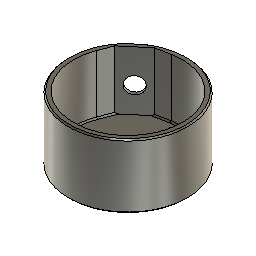
Gauge (Autodesk Fusion 360 design; units mm, degrees)
Autodesk Fusion 360 part; units mm, degrees
sketch "Sketch1" plane through (0, 0, 0) normal (0, 0, 1) x (1, 0, 0)
  circle A0 centre (0, 0) radius 42.5
  circle A1 centre (0, 0) radius 46.5
  dimension "d1" = 85
  dimension "d2" = 93
  constraint coincident A0.centre A1.centre
  constraint concentric A0 A1
  measures "d1" diameter of A0
  measures "d2" diameter of A1
extrude "Extrude1" add sketch "Sketch1" along normal blind 46 makes body 1
extrude "Extrude2" add sketch "Sketch1" against normal blind 4 contours A0 | A1 bodies 1
ref_plane "WorkPlane1" through (0, 0, 46) normal (0, 0, 1) x (1, 0, 0)
sketch "Sketch3" plane through (0, 0, 46) normal (0, 0, 1) x (1, 0, 0)
  circle A0 centre (0, 0) radius 46.5
  circle A1 centre (0, 0) radius 42.5
  circle A2 centre (0, 0) radius 49
  circle A3 centre (0, 0) radius 40.5
  circle A4 centre (0, 0) radius 46.9
  dimension "d9" = 98
  dimension "d10" = 81
  dimension "d50" = 0.4
  constraint concentric A0 A2
  constraint concentric A0 A3
  measures "d9" diameter of A2
  measures "d10" diameter of A3
extrude "Extrude3" add sketch "Sketch3" along normal blind 4 separate body contours A0 | A1 | A2 | A4 makes body 2
extrude "Extrude4" add sketch "Sketch3" against normal blind 12 contours A2 bodies 2
chamfer "Chamfer1" distance 3 angle 45 1 edges at (-37.7593, 14.6454, 50) on bodies 2
chamfer "Chamfer2" distance 2 angle 65 1 edges at (-45.684, -17.7192, 50) measured on face at (46.8223, -4.5955, 50) on bodies 2
chamfer "Chamfer3" distance 1 angle 45 1 edges at (-45.684, 17.7192, 34) measured on face at (48.1176, -2.4344, 34) on bodies 2
chamfer "Chamfer4" distance 1 angle 45 1 edges at (-43.3532, 16.8151, -4) measured on face at (10.204, -8.5364, -4) on bodies 1
ref_plane "WorkPlane2" through (0, 0, 0) normal (0, 0, -1) x (-1, 0, 0)
sketch "Sketch4" plane through (0, 0, 0) normal (0, 0, -1) x (1, 0, 0)
  circle A0 centre (0, 0) radius 46.5 construction
  line L0 (-37.4678, -27.5394) -> (-20.6148, -41.6807)
  line L1 (-20.6148, -41.6807) -> (-26.0712, -48.1834)
  line L2 (-26.0712, -48.1834) -> (-42.9242, -34.0421)
  line L3 (-42.9242, -34.0421) -> (-37.4678, -27.5394)
  line L4 (0, 0) -> (-58.0825, -69.2201) construction
  line L5 (-18.892, -39.6276) -> (-35.745, -25.4862)
  circle A1 centre (0, 0) radius 42.5
  line L6 (-18.892, -39.6276) -> (-8.0933, -41.7223)
  line L7 (-35.745, -25.4862) -> (-39.683, -15.2153)
  line L8 (-39.683, -15.2153) -> (-8.0933, -41.7223)
  line L9 (0, 0) -> (-65, 0) construction
  dimension "d26" = 22
  dimension "d58" = 50
  constraint coincident A0 L0.start
  constraint coincident A0 L0.end
  constraint coincident A0.centre L4.start
  constraint midpoint L0 L4
  constraint perpendicular L4 L5
  constraint tangent L5 A1
  constraint coincident A1 L6.end
  constraint coincident A1 L7.end
  constraint tangent A1 L6
  constraint tangent A1 L7
  constraint perpendicular L0 L3
  constraint perpendicular L0 L1
  constraint parallel L0 L2
  constraint horizontal L9
  constraint coincident L3 L5.end
  constraint coincident L1 L5.start
  measures "d26" distance of L0.start L0.end
  measures "d58" angle of L4 L9
extrude "Extrude5" cut sketch "Sketch4" along normal through all and the other way through all contours L0 L1 L2 L3 bodies 1
sketch "Sketch5" plane through (-29.0413, 34.61, 0) normal (-0.642788, 0.766044, 0) x (-0.766044, -0.642788, 0)
  line L0 (-11, 46) -> (-11, -3)
  circle A0 centre (0, 20) radius 6.5
  line L1 (11, 46) -> (-11, 46)
  spline S0 degree 2 poles (-5.3852, -4) (-8.1621, -3.6713) (-11, -3) knots 0 0 0 0.570553 0.570553 0.570553 weights 1 1.001868 1
  line L2 (-5.3852, -4) -> (5.3852, -4)
  spline S1 degree 2 poles (11, -3) (8.1621, -3.6713) (5.3852, -4) knots 0 0 0 0.570553 0.570553 0.570553 weights 1 1.001868 1
  line L3 (11, -3) -> (11, 46)
  line L4 (-11, 0) -> (11, 0)
  dimension "d30" = 13
  dimension "d61" = 20
  dimension "d62" = 11
  measures "d30" diameter of A0
  measures "d61" distance of A0.centre L4
  measures "d62" distance of L0 A0.centre
extrude "Extrude6" cut sketch "Sketch5" against normal blind 15 contours A0 bodies 1
sketch "Sketch6" plane through (0, 0, 0) normal (0, 0, 1) x (-1, 0, 0)
  circle A0 centre (0, -35) radius 3
  circle A1 centre (30.31, 17.5) radius 3
  circle A2 centre (-30.31, 17.5) radius 3
  circle A3 centre (0, 0) radius 5
  circle A4 centre (0, 0) radius 42.5
  circle A5 centre (20, 0) radius 2.75
  line L0 (0, 0) -> (65, 0)
  circle A6 centre (-20, 0) radius 2.75
  circle A7 centre (20, 0) radius 5
  circle A8 centre (-20, 0) radius 5
  dimension "d33" = 6
  dimension "d34" = 6
  dimension "d35" = 6
  dimension "d36" = 35
  dimension "d37" = 17.5
  dimension "d38" = 17.5
  dimension "d39" = 30.31
  dimension "d40" = 30.31
  dimension "d42" = 10
  dimension "d63" = 5.5
  dimension "d64" = 5.5
  dimension "d65" = 10
  dimension "d66" = 10
  dimension "d67" = 20
  dimension "d68" = 20
  constraint vertical A3.centre A0.centre
  constraint coincident A3.centre A4.centre
  constraint coincident A5.centre L0
  constraint concentric A5 A7
  constraint concentric A6 A8
  constraint horizontal A3.centre A6.centre
  measures "d33" diameter of A1
  measures "d34" diameter of A2
  measures "d35" diameter of A0
  measures "d36" distance of A3.centre A0.centre
  measures "d37" vertical distance of A3.centre A1.centre
  measures "d38" vertical distance of A3.centre A2.centre
  measures "d39" horizontal distance of A3.centre A2.centre
  measures "d40" horizontal distance of A3.centre A1.centre
  measures "d42" diameter of A3
  measures "d63" diameter of A6
  measures "d64" diameter of A5
  measures "d65" diameter of A8
  measures "d66" diameter of A7
  measures "d67" distance of A3.centre A5.centre
  measures "d68" distance of A3.centre A6.centre
extrude "Extrude7" cut sketch "Sketch6" against normal through all contours A3 | A5 L0 | A5 L0 | A6 bodies 1
extrude "Extrude8" add sketch "Sketch6" along normal blind 2 contours A0 | A1 | A2 bodies 1
sketch "Sketch7" plane through (0, 0, 2) normal (0, 0, 1) x (-1, 0, 0)
  circle A0 centre (0, -35) radius 3
  circle A1 centre (0, -35) radius 1.5
  circle A2 centre (30.31, 17.5) radius 1.5
  circle A3 centre (-30.31, 17.5) radius 1.5
  point P0 (30.31, 17.5)
  point P1 (-30.31, 17.5)
  dimension "d45" = 3
  dimension "d46" = 3
  dimension "d47" = 3
  constraint concentric A0 A1
  constraint coincident P0 A2.centre
  constraint coincident P1 A3.centre
  measures "d45" diameter of A1
  measures "d46" diameter of A2
  measures "d47" diameter of A3
extrude "Extrude9" cut sketch "Sketch7" against normal through all contours A1 | A2 | A3 bodies 1
chamfer "Chamfer5" distance 1 angle 45 1 edges at (-43.3532, -16.8151, 46) measured on face at (-19.1306, 39.3496, 46) on bodies 1
extrude "Extrude11" cut sketch "Sketch4" against normal through all contours L5 A1 L6 | L5 A1 L7 bodies 1
chamfer "Chamfer7" distance 1 angle 45 3 edges at (-13.4926, 40.6749, 0) (27.3185, -32.5569, 0) (-37.714, 20.3508, 0) on bodies 1
extrude "Extrude12" cut sketch "Sketch6" against normal blind 2 contours A5 L0 A7 | A5 L0 A7 | A8 bodies 1
chamfer "Chamfer8" distance 1 angle 45 2 edges at (-15.3384, -1.8081, 0) (24.6616, -1.8081, 0) on bodies 1
hidden bodies 2
named bodies: "Housing", "Surround"
